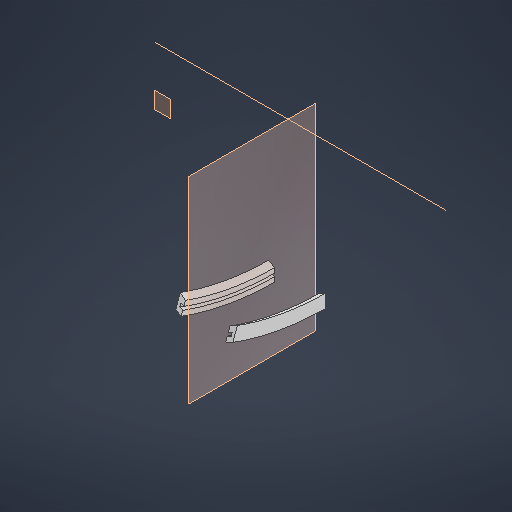
# Autodesk Inventor part: крепл направления
Saved by Autodesk Inventor 2026.2 (Build 302298000, 298)
## iProperties
Created: 2025-11-28
Part Number: крепл направления
Material: Типовые
Document SubType Name: Modeling
Designer: Phantom
Density: 1 g/cm^3
Appearance: По умолчанию
Author: Phantom
Autodesk Inventor part; units mm, degrees
ref_plane "XZ Plane" through (0, 0, 0) normal (0, 1, 0) x (-1, 0, 0)
sketch "Эскиз1" plane through (0, 0, 0) normal (0, 0, 1) x (1, 0, 0)
  arc A0 (74.5189, -162) -> (127.4811, -162) centre (101, -101) ccw
  arc A1 (48.4714, -162) -> (153.5286, -162) centre (101, -101) ccw
  line L0 (-97.5257, 0) -> (307.6841, 0) projected
  line L1 (-39.6386, -162) -> (244.9538, -162)
  line L2 (101, -167.5) -> (101, -181.5)
  arc A2 (142.003, -162) -> (59.997, -162) centre (101, -101) ccw
  circle A3 centre (101, -101) radius 72
  circle A4 centre (101, -101) radius 75
  line L3 (170.7391, -120.21) -> (170.39, -120.21)
  line L4 (170.39, -120.21) -> (173.4981, -120.21)
  line L5 (31.61, -120.21) -> (28.5019, -120.21)
  line L6 (74.5189, -162) -> (74.5189, -177.0197)
  line L7 (127.4811, -162) -> (127.4811, -177.0197)
  line L8 (70.5189, -166.2296) -> (70.5189, -169.5266)
  line L9 (131.4811, -166.2296) -> (131.4811, -169.5266)
  point P0 (0, 0)
  point P1 (167.5699, -124.21)
  point P2 (163.3181, -124.21)
  point P3 (38.6819, -124.21)
  point P4 (34.4301, -124.21)
  point P5 (101, -174.5)
  point P6 (57.3652, -162)
  point P7 (144.6348, -162)
  point P8 (62.7508, -162)
  point P9 (170.7391, -120.21)
  point P10 (74.5189, -167.9533)
  point P11 (74.5189, -171.1694)
  point P12 (127.4811, -171.1694)
  point P13 (127.4811, -167.9533)
  dimension "d0" = 133
  dimension "d1" = 161
  dimension "d3" = -101
  dimension "d4" = 61
  dimension "d30" = 1.5
  dimension "d31" = 1.5
  dimension "d33" = 73.5
  dimension "d34" = 4
  constraints: 17 point on circle, 16 end point, 5 centre point, 4 symmetric about line, 3 vertical, 2 coincident, 2 midpoint, 1 horizontal, 12 other
  measures "d0" diameter of A0
  measures "d1" diameter of A1
  measures "d3" distance from line of A1.centre L0
  measures "d30" radial gap between concentric circles of A2 A3
  measures "d31" radial gap between concentric circles of A2 A4
  measures "d33" radius of A2
  measures "d34" distance between parallel lines of L6 L8
ref_plane "РабПлоскость1" through (0, 0, 60) normal (0, 0, 1) x (1, 0, 0)
sketch "Эскиз2" plane through (0, 0, 60) normal (0, 0, 1) x (1, 0, 0)
  circle A0 centre (101, -101) radius 70.5
  line L0 (-96.1046, 0) -> (307.4472, 0) projected
  arc A1 (34.4301, -164.21) -> (167.5699, -164.21) centre (101, -141) ccw
  arc A2 (38.6819, -164.21) -> (163.3181, -164.21) centre (101, -141) ccw
  line L1 (-38.4543, -164.21) -> (249.797, -164.21)
  point P0 (0, 0)
  dimension "d9" = 141
  dimension "d10" = 141
  dimension "d11" = 133
  dimension "d12" = 23.21
  constraints: 4 point on circle, 4 point on line, 3 centre point, 2 end point, 1 coincident, 1 horizontal
  measures "d9" diameter of A1
  measures "d10" distance from line of L0 A1.centre
  measures "d11" diameter of A2
  measures "d12" distance from line of A1.centre L1
sketch "Эскиз3" plane through (0, 0, 0) normal (1, 0, 0) x (0, 1, 0)
  arc A0 (-211.5, 60) -> (-171.5, 0) centre (-52.4181, 122.7213) ccw
  point P0 (0, 0)
  point P1 (-164.21, 60)
  point P2 (-162, 0)
  dimension "d13" = 171
  constraints: 2 point on circle, 1 centre point
  measures "d13" radius of A0
sketch "Эскиз4" plane through (0, 0, 0) normal (1, 0, 0) x (0, 1, 0)
  line L0 (0, -518.9739) -> (0, 512.8159) projected
  arc A0 (-151.3766, 110.2381) -> (-171.5, 0) centre (155.0612, -2.6563) ccw
  arc A1 (-171.3994, 5.874) -> (-171.5, 0) centre (0, 0) ccw
  point P0 (-131.3766, -110.2381)
  dimension "d25" = 326.572
  constraints: 5 point on circle, 2 centre point, 1 coincident
  measures "d25" radius of A0
sweep "Сдвиг2" add profiles "Эскиз1" path "Эскиз4" path curves A0 contours A0 L2 A3 L6 | A0 L7 A3 L2 | L6 A4 L8 A3 | A3 L2 A4 L6 | A3 L7 A4 L2 | A3 L9 A4 L7 | A4 L2 A1 L6 | A4 L7 A1 L2
ref_plane "РабПлоскость2" through (101, 0, 0) normal (1, 0, 0) x (0, 1, 0)
sketch "Эскиз5" plane through (101, 0, 0) normal (1, 0, 0) x (0, 1, 0)
  line L0 (-177.0197, 0) -> (-177.0197, 0) projected
  line L1 (-156.5714, 112.104) -> (-156.5714, 112.104) projected
  line L2 (-177.0197, 0) -> (-177.0197, 0) projected
  line L3 (-156.5714, 112.104) -> (-156.5714, 112.104) projected
  arc A0 (-162, 0) -> (-142.4359, 107.0266) centre (155.0612, -2.6563) ccw projected
  line L4 (-162, 0) -> (-181.5, 0) projected
  circle A1 centre (155.0612, -2.6563) radius 336.5717
  arc A2 (-156.5714, 112.104) -> (-177.0197, 0) centre (155.0612, -2.6563) ccw projected
  arc A3 (-156.5714, 112.104) -> (-177.0197, 0) centre (155.0612, -2.6563) ccw projected
  arc A4 (-156.5714, 112.104) -> (-177.0197, 0) centre (155.0612, -2.6563) ccw projected
  arc A5 (-156.5714, 112.104) -> (-177.0197, 0) centre (155.0612, -2.6563) ccw projected
  point P0 (0, 0)
  point P1 (-162, 0)
  point P2 (-142.4359, 107.0266)
  point P3 (-162, 0)
  point P4 (-142.4359, 107.0266)
  dimension "d28" = 673.1434
  constraints: 1 coincident, 3 other
sketch "Эскиз7" plane through (101, -101, 0) normal (0, 0, -1) x (-1, 0, 0)
  arc A0 (26.4811, -66.9533) -> (30.4811, -65.2296) centre (0, 0) ccw projected
  line L0 (26.4811, -61) -> (26.4811, -66.9533) projected
  arc A1 (-26.4811, -61) -> (26.4811, -61) centre (0, 0) ccw projected
  line L1 (-26.4811, -66.9533) -> (-26.4811, -61) projected
  arc A2 (-30.4811, -65.2296) -> (-26.4811, -66.9533) centre (0, 0) ccw projected
  line L2 (-30.4811, -68.5266) -> (-30.4811, -65.2296) projected
  arc A3 (-30.4811, -68.5266) -> (-26.4811, -70.1694) centre (0, 0) ccw projected
  line L3 (-26.4811, -76.0197) -> (-26.4811, -70.1694) projected
  arc A4 (-26.4811, -76.0197) -> (26.4811, -76.0197) centre (0, 0) ccw projected
  line L4 (26.4811, -70.1694) -> (26.4811, -76.0197) projected
  arc A5 (26.4811, -70.1694) -> (30.4811, -68.5266) centre (0, 0) ccw projected
  line L5 (30.4811, -65.2296) -> (30.4811, -68.5266) projected
  line L6 (-26.6811, -66.6585) -> (-26.6811, -60.6944)
  arc A6 (-26.6811, -60.6944) -> (26.6811, -60.6944) centre (0, 0) ccw
  line L7 (26.6811, -60.6944) -> (26.6811, -66.6585)
  arc A7 (26.6811, -66.6585) -> (30.6811, -64.9146) centre (0, 0) ccw
  line L8 (30.6811, -64.9146) -> (30.6811, -68.6565)
  arc A8 (26.6811, -70.3076) -> (30.6811, -68.6565) centre (0, 0) ccw
  line L9 (26.6811, -70.3076) -> (26.6811, -76.1617)
  arc A9 (-26.6811, -76.1617) -> (26.6811, -76.1617) centre (0, 0) ccw
  line L10 (-26.6811, -76.1617) -> (-26.6811, -70.3076)
  arc A10 (-30.6811, -68.6565) -> (-26.6811, -70.3076) centre (0, 0) ccw
  line L11 (-30.6811, -68.6565) -> (-30.6811, -64.9146)
  arc A11 (-30.6811, -64.9146) -> (-26.6811, -66.6585) centre (0, 0) ccw
  circle A12 centre (0, 0) radius 66.5
  line L12 (-34.1811, -57.043) -> (-34.1811, -72.8828)
  line L13 (-26.4811, -66.9533) -> (-26.4811, -61) projected
  circle A13 centre (0, 0) radius 80.5
  line L14 (34.1811, -57.043) -> (34.1811, -72.8828)
  point P0 (101, 101)
  point P1 (26.6811, -75.9498)
  point P2 (34.1811, -72.8828)
  point P3 (34.1811, -57.043)
  point P4 (26.6811, -60.9128)
  point P5 (-26.6811, -60.9128)
  point P6 (-26.6811, -75.9498)
  dimension "d35" = 0.2
  dimension "d36" = 3.5
  constraints: 16 end point, 12 point on circle, 6 centre point, 2 coincident, 1 parallel, 19 other
  measures "d35" radial gap between concentric circles of A2 A11
  measures "d36" distance between parallel lines of L12 L11
sketch3d "3D эскиз1"
  arc A0 (127.4811, -177.0197, 0) -> (127.4811, -156.5714, 112.104) centre (127.4811, 155.0612, -2.6563) ccw
sweep "Сдвиг3" add profiles "Эскиз7" path "3D эскиз1" contours A12 L14 A13 L9 A8 L8 A7 L7 | L6 A11 L11 A10 L10 A13 L12 A12
sketch "Эскиз8" plane through (101, -101, 0) normal (0, 0, -1) x (-1, 0, 0)
  arc A0 (26.4811, -66.9533) -> (30.4811, -65.2296) centre (0, 0) ccw projected
  line L0 (26.4811, -61) -> (26.4811, -66.9533) projected
  arc A1 (-26.4811, -61) -> (26.4811, -61) centre (0, 0) ccw projected
  line L1 (-26.4811, -66.9533) -> (-26.4811, -61) projected
  arc A2 (-30.4811, -65.2296) -> (-26.4811, -66.9533) centre (0, 0) ccw projected
  line L2 (-30.4811, -68.5266) -> (-30.4811, -65.2296) projected
  arc A3 (-30.4811, -68.5266) -> (-26.4811, -70.1694) centre (0, 0) ccw projected
  line L3 (-26.4811, -76.0197) -> (-26.4811, -70.1694) projected
  arc A4 (-26.4811, -76.0197) -> (26.4811, -76.0197) centre (0, 0) ccw projected
  line L4 (26.4811, -70.1694) -> (26.4811, -76.0197) projected
  arc A5 (26.4811, -70.1694) -> (30.4811, -68.5266) centre (0, 0) ccw projected
  line L5 (30.4811, -65.2296) -> (30.4811, -68.5266) projected
  point P0 (101, 101)
sketch3d "3D эскиз2"
  arc A0 (135.1811, -173.8828, 0) -> (135.1811, -153.6191, 111.0436) centre (135.1811, 155.0612, -2.6563) ccw
sweep "Сдвиг4" cut profiles "Эскиз8" path "3D эскиз2"
